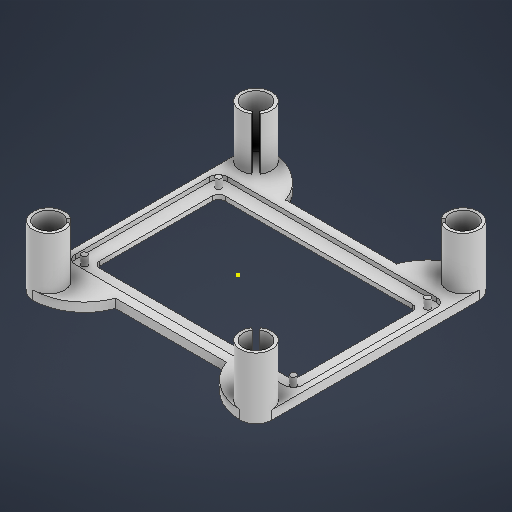
# Autodesk Inventor part: Drone
Saved by Autodesk Inventor 2026.2 (Build 302298000, 298)
## iProperties
Created: 2026-01-22
Part Number: Drone
Material: Ogólny
Document SubType Name: Modeling
Designer: DeathLock
Density: 1 g/cm^3
Appearance: Domyślna
Author: DeathLock
Autodesk Inventor part; units mm, degrees
ref_plane "YZ Plane" through (0, 0, 0) normal (1, 0, 0) x (0, 1, 0)
ref_plane "XZ Plane" through (0, 0, 0) normal (0, 1, 0) x (-1, 0, 0)
ref_plane "XY Plane" through (0, 0, 0) normal (0, 0, 1) x (1, 0, 0)
sketch "Szkic1" plane through (0, 0, 0) normal (0, 1, 0) x (-1, 0, 0)
  line L0 (33.7374, 40.303) -> (-46.2626, 40.303)
  line L1 (-46.2626, 40.303) -> (-46.2626, -39.697)
  line L2 (-46.2626, -39.697) -> (33.7374, -39.697)
  line L3 (33.7374, -39.697) -> (33.7374, 40.303)
  point P0 (0, 0)
  dimension "d0" = 80
  dimension "d1" = 80
  constraints: 8 end point, 2 parallel, 1 horizontal, 1 perpendicular
  measures "d0" distance of L2.end L0.start
  measures "d1" distance of L1.end L2.end
extrude "Wyciągnięcie proste1" add sketch "Szkic1" along normal blind 3
sketch "Szkic2" plane through (0, 3, 0) normal (0, 1, 0) x (1, 0, 0)
  line L0 (-33.7374, 39.697) -> (-33.7374, -40.303) projected
  line L1 (-33.7374, -0.303) -> (46.2626, -0.303)
  line L2 (46.2626, -40.303) -> (46.2626, 39.697) projected
  line L3 (-31.7374, -25.803) -> (44.2626, -25.803)
  line L4 (44.2626, -25.803) -> (44.2626, 25.197)
  line L5 (44.2626, 25.197) -> (-31.7374, 25.197)
  line L6 (-31.7374, 25.197) -> (-31.7374, -25.803)
  line L7 (-33.7374, -40.303) -> (46.2626, -40.303) projected
  line L8 (46.2626, 39.697) -> (-33.7374, 39.697) projected
  line L9 (-31.7374, -25.803) -> (-28.7374, -25.803)
  line L10 (-28.7374, -25.803) -> (-28.7374, -22.803)
  line L11 (-28.7374, -22.803) -> (-31.7374, -22.803)
  line L12 (-31.7374, -22.803) -> (-31.7374, -25.803)
  line L13 (-31.7374, 25.197) -> (-28.7374, 25.197)
  line L14 (-28.7374, 25.197) -> (-28.7374, 22.197)
  line L15 (-28.7374, 22.197) -> (-31.7374, 22.197)
  line L16 (-31.7374, 22.197) -> (-31.7374, 25.197)
  line L17 (44.2626, -25.803) -> (41.2626, -25.803)
  line L18 (41.2626, -25.803) -> (41.2626, -22.803)
  line L19 (41.2626, -22.803) -> (44.2626, -22.803)
  line L20 (44.2626, -22.803) -> (44.2626, -25.803)
  line L21 (44.2626, 25.197) -> (41.2626, 25.197)
  line L22 (41.2626, 25.197) -> (41.2626, 22.197)
  line L23 (41.2626, 22.197) -> (44.2626, 22.197)
  line L24 (44.2626, 22.197) -> (44.2626, 25.197)
  circle A0 centre (-28.7374, -22.803) radius 3
  circle A1 centre (-28.7374, 22.197) radius 3
  circle A2 centre (41.2626, 22.197) radius 3
  circle A3 centre (41.2626, -22.803) radius 3
  point P0 (0, 0)
  point P1 (6.2626, -25.803)
  point P2 (6.2626, 25.197)
  point P3 (-31.7374, -0.303)
  point P4 (44.2626, -0.303)
  dimension "d4" = 76
  dimension "d5" = 51
  dimension "d6" = 14.5
  dimension "d7" = 14.5
  dimension "d8" = 2
  dimension "d9" = 2
  dimension "d10" = 3
  dimension "d11" = 3
  dimension "d12" = 3
  dimension "d13" = 3
  dimension "d14" = 3
  dimension "d15" = 3
  dimension "d16" = 3
  dimension "d17" = 3
  constraints: 42 end point, 10 parallel, 6 midpoint, 5 horizontal, 5 perpendicular, 4 coincident, 12 other
  measures "d4" distance of L5.end L4.end
  measures "d5" distance of L4.end L3.end
  measures "d6" distance from line of L7 point (6.263, -25.803)
  measures "d7" distance from line of L8 point (6.263, 25.197)
  measures "d8" distance from line of L0 point (-31.737, -0.303)
  measures "d9" distance from line of L2 point (44.263, -0.303)
  measures "d10" distance of L11.end L10.end
  measures "d11" distance of L10.end L9.end
  measures "d12" distance of L14.end L15.end
  measures "d13" distance of L13.end L14.end
  measures "d14" distance of L18.end L19.end
  measures "d15" distance of L17.end L18.end
  measures "d16" distance of L23.end L22.end
  measures "d17" distance of L22.end L21.end
extrude "Wyciągnięcie proste2" cut sketch "Szkic2" against normal blind 1.5 contours L6 A1 L5 A2 L4 L1 | L1 L4 A3 L3 A0 L6 | A1 L14 L15 | L15 L14 A1 | A0 L10 L11 | L11 L10 A0 | A3 L18 L19 | L19 L18 A3 | A2 L22 L23 | L23 L22 A2
sketch "Szkic3" plane through (0, 1.5, 0) normal (0, 1, 0) x (1, 0, 0)
  arc A0 (-31.7374, -22.803) -> (-28.7374, -25.803) centre (-28.7374, -22.803) ccw projected
  arc A1 (44.2626, 22.197) -> (41.2626, 25.197) centre (41.2626, 22.197) ccw projected
  line L0 (-28.7374, -25.803) -> (41.2626, -25.803)
  line L1 (41.2626, -25.803) -> (41.2626, 25.197)
  line L2 (41.2626, 25.197) -> (-28.7374, 25.197)
  line L3 (-28.7374, 25.197) -> (-28.7374, -25.803)
  line L4 (-31.7374, -22.803) -> (-31.7374, 22.197) projected
  line L5 (44.2626, 22.197) -> (-31.7374, 22.197)
  line L6 (-31.7374, 22.197) -> (-31.7374, -22.803)
  line L7 (-31.7374, -22.803) -> (44.2626, -22.803)
  line L8 (44.2626, -22.803) -> (44.2626, 22.197)
  circle A2 centre (-28.7374, -22.803) radius 1
  circle A3 centre (-28.7374, 22.197) radius 1
  circle A4 centre (41.2626, -22.803) radius 1
  circle A5 centre (41.2626, 22.197) radius 1
  point P0 (0, 0)
  dimension "d20" = 2
  dimension "d21" = 2
  dimension "d22" = 2
  dimension "d23" = 2
  constraints: 16 end point, 4 centre point, 4 parallel, 4 point on line, 2 coincident, 2 horizontal, 2 perpendicular
  measures "d20" diameter of A2
  measures "d21" diameter of A3
  measures "d22" diameter of A4
  measures "d23" diameter of A5
extrude "Wyciągnięcie proste3" add sketch "Szkic3" along normal blind 3 contours A2 L3 L7 | L7 L3 A2 | L3 L7 A2 | A3 L3 L5 | L5 L3 A3 | L3 A2 L7 | A4 L7 L1 | L1 L7 A4 | L5 A3 L3 | L3 A3 L5 | L7 A4 L1 | L1 A4 L7 | A5 L1 L5 | L5 L1 A5 | L1 L5 A5 | L1 A5 L5
sketch "Szkic4" plane through (0, 3, 0) normal (0, 1, 0) x (1, 0, 0)
  line L0 (-33.7374, -40.303) -> (46.2626, -40.303) projected
  line L1 (46.2626, -40.303) -> (46.2626, 39.697) projected
  line L2 (-33.7374, -40.303) -> (46.2626, -40.303)
  line L3 (46.2626, -40.303) -> (46.2626, -29.703)
  line L4 (46.2626, -29.703) -> (-33.7374, -29.703)
  line L5 (-33.7374, -29.703) -> (-33.7374, -40.303)
  line L6 (46.2626, 39.697) -> (-33.7374, 39.697) projected
  line L7 (-33.7374, 39.697) -> (46.2626, 39.697)
  line L8 (46.2626, 39.697) -> (46.2626, 29.097)
  line L9 (46.2626, 29.097) -> (-33.7374, 29.097)
  line L10 (-33.7374, 29.097) -> (-33.7374, 39.697)
  line L11 (-33.7374, 39.697) -> (-33.7374, -40.303) projected
  line L12 (-33.7374, 34.397) -> (46.2626, 34.397)
  line L13 (46.2626, 34.397) -> (46.2626, -35.003)
  line L14 (46.2626, -35.003) -> (-33.7374, -35.003)
  line L15 (-33.7374, -35.003) -> (-33.7374, 34.397)
  line L16 (-33.7374, 39.697) -> (-28.4374, 39.697)
  line L17 (-28.4374, 39.697) -> (-28.4374, -40.303)
  line L18 (-28.4374, -40.303) -> (-33.7374, -40.303)
  line L19 (-33.7374, -40.303) -> (-33.7374, 39.697)
  line L20 (46.2626, -40.303) -> (40.9626, -40.303)
  line L21 (40.9626, -40.303) -> (40.9626, 39.697)
  line L22 (40.9626, 39.697) -> (46.2626, 39.697)
  line L23 (46.2626, 39.697) -> (46.2626, -40.303)
  circle A0 centre (-28.4374, 34.397) radius 5.3
  circle A1 centre (40.9626, 34.397) radius 5.3
  circle A2 centre (40.9626, -35.003) radius 5.3
  circle A3 centre (-28.4374, -35.003) radius 5.3
  line L24 (-28.4374, -35.003) -> (-24.6897, -31.2554)
  line L25 (-28.4374, -35.003) -> (-23.1374, -35.003) construction
  line L26 (-28.4374, -35.003) -> (-25.4928, -30.5962)
  line L27 (-28.4374, -35.003) -> (-23.1374, -35.003) construction
  line L28 (-28.4374, -35.003) -> (-24.0306, -32.0585)
  line L29 (-28.4374, -35.003) -> (-23.1374, -35.003) construction
  line L30 (40.9626, -35.003) -> (37.215, -31.2554)
  line L31 (40.9626, -35.003) -> (46.2626, -35.003) construction
  line L32 (40.9626, -35.003) -> (36.5558, -32.0585)
  line L33 (40.9626, -35.003) -> (46.2626, -35.003) construction
  line L34 (40.9626, -35.003) -> (38.0181, -30.5962)
  line L35 (40.9626, -35.003) -> (46.2626, -35.003) construction
  line L36 (-28.4374, 34.397) -> (-24.6897, 30.6493)
  line L37 (-28.4374, 34.397) -> (-24.0306, 31.4524)
  line L38 (-28.4374, 34.397) -> (-23.1374, 34.397) construction
  line L39 (-28.4374, 34.397) -> (-25.4928, 29.9902)
  line L40 (-28.4374, 34.397) -> (-23.1374, 34.397) construction
  line L41 (40.9626, 34.397) -> (37.215, 30.6493)
  line L42 (40.9626, 34.397) -> (36.5558, 31.4524)
  line L43 (40.9626, 34.397) -> (46.2626, 34.397) construction
  line L44 (40.9626, 34.397) -> (38.0181, 29.9902)
  line L45 (40.9626, 34.397) -> (46.2626, 34.397) construction
  circle A4 centre (-28.4374, 34.397) radius 4.3
  circle A5 centre (40.9626, 34.397) radius 4.3
  circle A6 centre (40.9626, -35.003) radius 4.3
  circle A7 centre (-28.4374, -35.003) radius 4.3
  point P0 (0, 0)
  point P1 (-26.0484, -31.4277)
  point P2 (-24.8621, -32.6141)
  point P3 (38.5737, -31.4277)
  point P4 (37.3873, -32.6141)
  point P5 (38.5737, 30.8217)
  point P6 (37.3873, 32.008)
  point P7 (-26.0484, 30.8217)
  point P8 (-24.8621, 32.008)
  dimension "d26" = 10.6
  dimension "d27" = 80
  dimension "d28" = 10.6
  dimension "d29" = 5.3
  dimension "d30" = 5.3
  dimension "d31" = 5.3
  dimension "d32" = 5.3
  dimension "d33" = 5.3
  dimension "d34" = 5.3
  dimension "d35" = 45
  dimension "d36" = 56.25
  dimension "d37" = 33.75
  dimension "d38" = 135
  dimension "d39" = 146.25
  dimension "d40" = 123.75
  dimension "d41" = 5.3
  dimension "d42" = 33.75
  dimension "d43" = 56.25
  dimension "d44" = 5.3
  dimension "d45" = 146.25
  dimension "d46" = 123.75
  dimension "d47" = 8.6
  dimension "d48" = 8.6
  dimension "d49" = 8.6
  dimension "d50" = 8.6
  constraints: 84 end point, 15 horizontal, 13 point on line, 12 point on circle, 10 equal length, 10 parallel, 8 centre point, 5 perpendicular, 4 coincident, 1 midpoint
  measures "d26" distance of L3.end L2.end
  measures "d27" distance of L8.end L9.end
  measures "d28" distance of L7.end L8.end
  measures "d29" distance between parallel lines of L4 L14
  measures "d30" distance between parallel lines of L0 L14
  measures "d31" distance between parallel lines of L12 L6
  measures "d32" distance between parallel lines of L12 L9
  measures "d33" distance of L17.end L18.end
  measures "d34" distance of L21.end L22.end
  measures "d35" angle of L25 L24
  measures "d36" angle of L27 L26
  measures "d37" angle of L29 L28
  measures "d38" angle of L31 L30
  measures "d39" angle of L33 L32
  measures "d40" angle of L35 L34
  measures "d41" distance of L36.start L37.end
  measures "d42" angle of L37 L38
  measures "d43" angle of L39 L40
  measures "d44" distance of L41.start L42.end
  measures "d45" angle of L42 L43
  measures "d46" angle of L44 L45
  measures "d47" diameter of A4
  measures "d48" diameter of A5
  measures "d49" diameter of A6
  measures "d50" diameter of A7
extrude "Wyciągnięcie proste4" add sketch "Szkic4" along normal blind 17.5 contours A3 L14 A7 L17 | L17 A7 L14 A3 | A3 L17 A7 L14 | A2 L14 A6 L21 | L21 A6 L14 A2 | L14 A7 L28 A3 | A3 L26 A7 L17 | L14 A6 L21 A2 | A2 L32 A6 L14 | L21 A6 L34 A2 | A0 L12 A4 L17 | L17 A4 L39 A0 | A0 L17 A4 L12 | A1 L44 A5 L21 | L21 A5 L12 A1 | A0 L12 A4 L17 | L12 A5 L21 A1 | L21 A5 L12 A1 | A0 L37 A4 L12 | L12 A5 L42 A1
sketch "Szkic5" plane through (0, 3, 0) normal (0, 1, 0) x (1, 0, 0)
  line L0 (-33.7374, -35.003) -> (-33.7374, -40.303) projected
  arc A0 (-25.4928, -30.5962) -> (-24.0306, -32.0585) centre (-28.4374, -35.003) ccw projected
  line L1 (-33.7374, -40.303) -> (46.2626, -40.303) projected
  line L2 (46.2626, -40.303) -> (40.9626, -35.003)
  line L3 (46.2626, -40.303) -> (53.758, -40.303) construction
  line L4 (-28.4374, 39.697) -> (-33.7374, 39.697) projected
  line L5 (-33.7374, 39.697) -> (-28.4374, 34.397)
  line L6 (46.2626, 39.697) -> (40.9626, 34.397)
  line L7 (-33.7374, -40.303) -> (-28.4374, -35.003)
  circle A1 centre (-28.4374, 34.397) radius 5.3
  circle A2 centre (40.9626, 34.397) radius 5.3
  circle A3 centre (40.9626, -35.003) radius 5.3
  circle A4 centre (-28.4374, -35.003) radius 5.3
  line L8 (-33.7374, 39.697) -> (-33.7374, 34.397)
  line L9 (46.2626, 39.697) -> (40.9626, 39.697)
  line L10 (46.2626, 39.697) -> (46.2626, 34.397)
  line L11 (46.2626, -40.303) -> (46.2626, -35.003)
  line L12 (46.2626, -40.303) -> (46.2626, -35.003) projected
  point P0 (0, 0)
  point P1 (-28.4374, -40.303)
  point P2 (40.9626, -40.303)
  dimension "d53" = 135
  constraints: 19 end point, 4 coincident, 2 centre point, 2 point on circle, 1 concentric, 1 equal length, 1 horizontal, 1 perpendicular, 1 tangent, 1 vertical, 6 other
  measures "d53" angle of L3 L2
extrude "Wyciągnięcie proste5" cut sketch "Szkic5" against normal blind 17.5 contours A0 L7 L0 | L7 A0 L1 | A3 L2 L1 | L2 A3 L11 | A1 L5 L4 | L5 A1 L8 | L10 A2 L6 | L6 A2 L9
sketch "Szkic6" plane through (0, 1.5, 0) normal (0, 1, 0) x (1, 0, 0)
  point P0 (0, 0)
sketch "Szkic7" plane through (0, 1.5, 0) normal (0, 1, 0) x (1, 0, 0)
  arc A0 (-31.7374, -22.803) -> (-28.7374, -25.803) centre (-28.7374, -22.803) ccw projected
  line L0 (44.2626, 22.197) -> (44.2626, -22.803) projected
  line L1 (-31.7374, -22.803) -> (44.2626, -22.803)
  line L2 (44.2626, -22.803) -> (44.2626, 22.197)
  line L3 (44.2626, 22.197) -> (-31.7374, 22.197)
  line L4 (-31.7374, 22.197) -> (-31.7374, -22.803)
  arc A1 (44.2626, 22.197) -> (41.2626, 25.197) centre (41.2626, 22.197) ccw projected
  line L5 (41.2626, 25.197) -> (-28.7374, 25.197)
  line L6 (-28.7374, 25.197) -> (-28.7374, -25.803)
  line L7 (-28.7374, -25.803) -> (41.2626, -25.803)
  line L8 (41.2626, -25.803) -> (41.2626, 25.197)
  line L9 (-28.7374, -22.803) -> (-26.6161, -20.6817)
  line L10 (-28.7374, -22.803) -> (-25.7374, -22.803) construction
  line L11 (41.2626, 22.197) -> (39.1413, 20.0756)
  line L12 (41.2626, -22.803) -> (39.1413, -20.6817)
  circle A2 centre (-28.7374, 22.197) radius 1 projected
  line L13 (-28.7374, 22.197) -> (-26.6161, 20.0756)
  line L14 (-26.6161, -20.6817) -> (39.1413, -20.6817)
  line L15 (39.1413, -20.6817) -> (39.1413, 20.0756)
  line L16 (39.1413, 20.0756) -> (-26.6161, 20.0756)
  line L17 (-26.6161, 20.0756) -> (-26.6161, -20.6817)
  line L18 (-26.6161, -20.6817) -> (-25.1163, -19.1819)
  circle A3 centre (-25.1163, -19.1819) radius 2.121
  line L19 (-26.6161, 20.0756) -> (-25.1163, 18.5759)
  line L20 (39.1413, 20.0756) -> (37.6415, 18.5759)
  line L21 (39.1413, -20.6817) -> (37.6415, -19.1819)
  circle A4 centre (-25.1163, 18.5759) radius 2.121
  circle A5 centre (37.6415, 18.5759) radius 2.121
  circle A6 centre (37.6415, -19.1819) radius 2.121
  line L22 (37.6415, -21.3029) -> (-25.1163, -21.3029)
  line L23 (-25.1163, -21.3029) -> (-25.1163, 20.6969)
  line L24 (-25.1163, 20.6969) -> (37.6415, 20.6969)
  line L25 (37.6415, 20.6969) -> (37.6415, -21.3029)
  line L26 (-27.2373, 18.5759) -> (39.7625, 18.5759)
  line L27 (39.7625, 18.5759) -> (39.7625, -19.1819)
  line L28 (39.7625, -19.1819) -> (-27.2373, -19.1819)
  line L29 (-27.2373, -19.1819) -> (-27.2373, 18.5759)
  point P0 (0, 0)
  dimension "d56" = 3
  dimension "d57" = 45
  dimension "d58" = 3
  dimension "d59" = 3
  dimension "d60" = 3
  dimension "d61" = 2.121
  dimension "d62" = 2.121
  dimension "d63" = 2.121
  dimension "d64" = 2.121
  constraints: 58 end point, 10 parallel, 6 horizontal, 6 point on circle, 5 perpendicular, 4 coincident, 2 centre point, 2 point on line, 1 equal length, 6 other
  measures "d56" distance of L9.start L9.end
  measures "d57" angle of L10 L9
  measures "d58" distance of L11.start L11.end
  measures "d59" distance of L12.start L12.end
  measures "d60" distance of L13.start L13.end
  measures "d61" distance of L9.end L18.end
  measures "d62" distance of L16.end L19.end
  measures "d63" distance of L11.end L20.end
  measures "d64" distance of L14.end L21.end
extrude "Wyciągnięcie proste6" cut sketch "Szkic7" against normal blind 17.5 contours L18 L23 L14 | A3 L28 L17 | L17 L28 L18 | L14 L23 A3 | A6 L25 L14 | L21 L28 L15 | L14 L25 L21 | L15 L28 A6 | L23 L28 A3 L14 | L14 A3 L23 | L28 A3 L17 | L17 A3 L23 L28 | L23 A3 L28 | L29 A4 L17 A3 | A3 L14 A6 L22 | A5 L26 L15 | L20 L25 L16 | L15 L26 L20 | L16 L25 A5 | L25 A6 L14 | L14 A6 L28 L25 | L28 L25 A6 L15 | L15 A6 L28 | L28 A6 L25 | A6 L15 A5 L27 | A4 L23 L16 | L19 L26 L17 | L16 L23 L19 | L17 L26 A4 | A3 L28 A6 L14 | L17 A4 L23 A3 | L23 A4 L26 A5 L25 A6 L28 A3 | L26 L17 A4 | L26 A5 L15 | L15 A5 L25 L26 | L25 L26 A5 L16 | L16 A5 L25 | L25 A5 L26 | A5 L16 A4 L24 | A6 L25 A5 L15 | L23 A4 L16 | L16 A4 L26 L23 | L26 L23 A4 L17 | L26 A4 L23 | A5 L26 A4 L16
sketch "Szkic8" plane through (0, 3, 0) normal (0, 1, 0) x (1, 0, 0)
  circle A0 centre (-28.7374, 22.197) radius 1 projected
  line L0 (40.9626, 39.697) -> (-28.4374, 39.697) projected
  arc A1 (-11.4868, 25.1563) -> (-28.4374, 39.697) centre (-28.7374, 22.197) ccw
  circle A2 centre (-28.7374, -22.803) radius 1 projected
  line L1 (-28.4374, -40.303) -> (40.9626, -40.303) projected
  arc A3 (-28.4374, -40.303) -> (-11.4936, -25.8018) centre (-28.7374, -22.803) ccw
  circle A4 centre (41.2626, -22.803) radius 1 projected
  arc A5 (36.5558, -32.0585) -> (40.9626, -40.303) centre (40.9626, -35.003) ccw projected
  arc A6 (24.0191, -25.8032) -> (40.9626, -40.303) centre (41.2626, -22.803) ccw
  arc A7 (40.9626, 39.697) -> (24.0191, 25.197) centre (41.2626, 22.197) ccw
  line L2 (41.2626, -25.803) -> (-28.7374, -25.803) projected
  line L3 (-28.7374, -25.803) -> (41.2626, -25.803)
  line L4 (41.2626, -25.803) -> (41.2626, -28.803)
  line L5 (41.2626, -28.803) -> (-28.7374, -28.803)
  line L6 (-28.7374, -28.803) -> (-28.7374, -25.803)
  line L7 (-28.7374, 25.197) -> (41.2626, 25.197) projected
  line L8 (41.2626, 25.197) -> (-28.7374, 25.197)
  line L9 (-28.7374, 25.197) -> (-28.7374, 28.197)
  line L10 (-28.7374, 28.197) -> (41.2626, 28.197)
  line L11 (41.2626, 28.197) -> (41.2626, 25.197)
  point P0 (0, 0)
  point P1 (-12.2954, 28.197)
  point P2 (24.8206, 28.197)
  point P3 (40.7021, -40.2966)
  point P4 (24.8206, -28.803)
  point P5 (-12.2954, -28.803)
  dimension "d67" = 3
  dimension "d68" = 3
  constraints: 16 end point, 8 point on circle, 4 centre point, 4 parallel, 3 coincident, 2 horizontal, 2 perpendicular, 1 point on line
  measures "d67" distance of L3.end L4.end
  measures "d68" distance of L8.end L9.end
extrude "Wyciągnięcie proste7" cut sketch "Szkic8" against normal blind 17.5 contours A7 L10 A1 L0 | A3 L5 A6 L1
